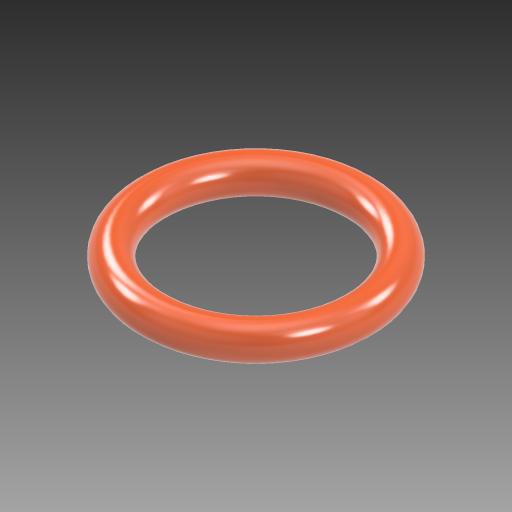
# Autodesk Inventor part: FRC 2024 Note
Saved by Autodesk Inventor 2024 (Build 280153000, 153)
## iProperties
Created: 2024-01-07
Part Number: FRC 2024 Note
Material: ABS Plastic
Document SubType Name: Modeling
Surface Area: 1528.19 cm^2
Volume: 1940.81 cm^3
Appearance: Smooth - Light Orange
Autodesk Inventor part; units mm, degrees
ref_plane "YZ Plane" through (0, 0, 0) normal (1, 0, 0) x (0, 1, 0)
ref_plane "XZ Plane" through (0, 0, 0) normal (0, 1, 0) x (-1, 0, 0)
ref_plane "XY Plane" through (0, 0, 0) normal (0, 0, 1) x (1, 0, 0)
sketch "Sketch1" plane through (0, 0, 0) normal (0, 0, 1) x (1, 0, 0)
  circle A0 centre (-152.4, 0) radius 25.4
  line L0 (0, 0) -> (0, 27.5858) construction
  dimension "d0" = 50.8
  dimension "d1" = 304.8
  constraints: 2 end point, 1 centre point, 1 horizontal alignment, 1 vertical
  measures "d0" diameter of A0
  measures "d1" diameter of A0.centre L0
revolve "Revolution1" add sketch "Sketch1" angle 360 about axis through (0, 0, 0) along (0, 1, 0)
body "Solid1"
